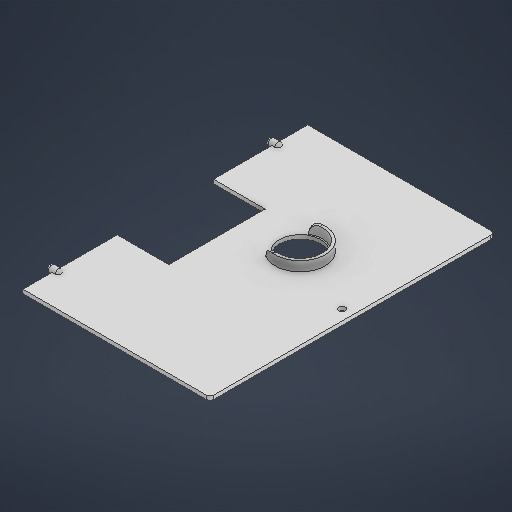
# Autodesk Inventor part: Base Shell Top V3
Saved by Autodesk Inventor 2026.2 (Build 302298000, 298)
## iProperties
Created: 2023-01-05
Part Number: Base Shell Top V3
Material: Generic
Document SubType Name: Modeling
Designer: vandj
Density: 1 g/cm^3
Appearance: Default
Author: vandj
Autodesk Inventor part; units mm, degrees
ref_plane "YZ Plane" through (0, 0, 0) normal (1, 0, 0) x (0, 1, 0)
ref_plane "XZ Plane" through (0, 0, 0) normal (0, 1, 0) x (-1, 0, 0)
ref_plane "XY Plane" through (0, 0, 0) normal (0, 0, 1) x (1, 0, 0)
sketch "Sketch1" plane through (0, 0, 0) normal (0, 1, 0) x (-1, 0, 0)
  line L0 (-48.571, 73.95) -> (48.571, 73.95)
  line L1 (48.571, 73.95) -> (48.571, -73.95)
  line L2 (48.571, -73.95) -> (-48.571, -73.95)
  line L3 (-48.571, -73.95) -> (-48.571, 73.95)
  line L4 (-48.571, 73.95) -> (48.571, -73.95) construction
  line L5 (48.571, 73.95) -> (-48.571, -73.95) construction
  circle A0 centre (-43.171, 0) radius 1.75
  line L6 (-48.571, -73.95) -> (-48.571, -59.45)
  circle A1 centre (-6.429, -15) radius 10.75
  line L7 (-67.9994, 0) -> (67.9994, 0) construction
  point P0 (0, 0)
  dimension "d0" = 97.142
  dimension "d1" = 147.9
  dimension "d3" = 3.5
  dimension "d54" = 55
  dimension "d61" = 5.4
  dimension "d62" = 15
  dimension "d63" = 21.5
  constraints: 14 end point, 2 centre point, 2 midpoint, 2 parallel, 2 point on line, 1 horizontal, 1 perpendicular
  measures "d0" distance of L1.end L2.end
  measures "d1" distance of L0.end L1.end
  measures "d3" diameter of A0
  measures "d54" distance from line of A1.centre L1
  measures "d61" distance from line of L3 A0.centre
  measures "d62" distance from line of L7 A1.centre
  measures "d63" diameter of A1
extrude "Lid Shape" add sketch "Sketch1" along normal blind 2
sketch "Sketch2" plane through (0, 2, 0) normal (0, 1, 0) x (1, 0, 0)
  circle A0 centre (6.429, 15) radius 10.75
  circle A1 centre (6.429, 15) radius 11.5
  circle A2 centre (6.429, 15) radius 13
  line L0 (6.429, 15) -> (-0.071, 3.7417)
  line L1 (6.429, 15) -> (19.429, 15) construction
  line L2 (6.429, 15) -> (-0.071, 26.2583)
  circle A3 centre (6.429, 15) radius 10.75 construction
  point P0 (0.679, 24.9593)
  point P1 (0.679, 5.0407)
  dimension "d64" = 26
  dimension "d65" = 23
  dimension "d66" = 120
  dimension "d67" = 120
  constraints: 6 end point, 3 centre point, 2 coincident, 2 concentric, 2 point on circle, 1 horizontal
  measures "d64" diameter of A2
  measures "d65" diameter of A1
  measures "d66" angle of L1 L2
  measures "d67" angle of L1 L0
extrude "Switch Protector" add sketch "Sketch2" along normal blind 5 contours L2 A2 L0 A1 picked at (18.7089, 13.1166)
fillet "Fillet1" radius 5 2 edges at (0.304, 7, -4.3912) (0.304, 7, -25.6088)
fillet "Fillet2" radius 2 2 edges at (48.571, 1, 73.95) (48.571, 1, -73.95)
sketch "Sketch4" plane through (-48.571, 0, -73.95) normal (-1, 0, 0) x (0, 0, 1)
  line L0 (16.95, 0) -> (16.95, 1.75) construction
  circle A0 centre (16.95, 1.75) radius 1.75
  circle A1 centre (73.95, 1.75) radius 1.75
  circle A2 centre (130.95, 1.75) radius 1.75
  line L1 (0, 2) -> (147.9, 2) projected
  line L2 (0, 0) -> (147.9, 0) projected
  line L3 (147.9, 0) -> (147.9, 2) projected
  line L4 (0, 2) -> (147.9, 2) projected
  line L5 (0, 0) -> (0, 2) projected
  line L6 (73.95, 4.2) -> (73.95, -0.7) construction
  point P0 (73.95, 0)
  dimension "d68" = 3.5
  dimension "d69" = 57
  dimension "d70" = 57
  constraints: 3 centre point, 3 tangent, 2 end point, 2 equal radius, 1 coincident, 1 midpoint
  measures "d68" diameter of A0
  measures "d69" distance from line of L0.end L6
  measures "d70" distance of A2.centre A1.centre
extrude "Peg Connectors" add sketch "Sketch4" along normal blind 3 and the other way blind 3 contours A0 L1 | L1 A0 | L1 A1 | A1 L1 | A2 L1 | A2 L1
fillet "Fillet5" radius 1.5 3 edges at (-45.571, 3.5, 57) (-45.571, 3.5, 0) (-45.571, 3.5, -57)
fillet "Fillet6" radius 1 3 edges at (-51.571, 1.75, 55.25) (-51.571, 1.75, -1.75) (-51.571, 1.75, -58.75)
sketch "Sketch7" plane through (0, 2, 0) normal (0, 1, 0) x (1, 0, 0)
  line L0 (-21.771, -25) -> (-21.771, 25)
  line L1 (-21.771, 25) -> (-55.771, 25)
  line L2 (-55.771, 25) -> (-55.771, -25)
  line L3 (-55.771, -25) -> (-21.771, -25)
  line L4 (-48.571, -1.7321) -> (-48.571, -55.2679) construction
  line L5 (-76.6394, 0) -> (69.4394, 0) construction
  point P0 (0, 0)
  dimension "d60" = 50
  dimension "d71" = 34
  dimension "d72" = 26.8
  constraints: 8 end point, 2 perpendicular, 1 other
  measures "d60" distance of L0.start L0.end
  measures "d71" distance of L0.end L1.end
  measures "d72" distance between parallel lines of L4 L0
extrude "Weapon Hole" cut sketch "Sketch7" along normal mid plane 6.7625
body "Solid1"
